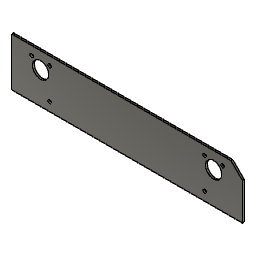
motor mount (Autodesk Fusion 360 design; units mm, degrees)
Autodesk Fusion 360 part; units mm, degrees
sketch "Sketch15" plane through (0, 0, 0) normal (0, 1, 0) x (1, 0, 0)
  line L0 (100, 21) -> (-100, 21)
  line L1 (-100, 21) -> (-100, -21)
  line L2 (-100, -21) -> (100, -21)
  line L3 (100, -21) -> (100, 21)
  line L4 (100, 21) -> (-100, -21) construction
  line L5 (-100, 21) -> (100, -21) construction
  dimension "d41" = 200
  dimension "d42" = 42
  constraint horizontal L0
  constraint perpendicular L0 L1
  constraint parallel L0 L2
  constraint parallel L1 L3
  constraint coincident L4 origin
  constraint coincident L5 origin
  measures "d41" distance of L1.end L2.end
  measures "d42" distance of L0.end L1.end
extrude "Extrude7" add sketch "Sketch15" along normal blind 1.5
hole "Hole5" at (67.2428, 0, 13.4085) direction (0, 1, 0) diameter 3 depth 7 tip angle 118
hole "Hole6" at (75.0009, 0, 6.5047) direction (0, 1, 0) diameter 14 depth 15 tip angle 118
hole "Hole7" at (82.7411, 0, 13.4378) direction (0, 1, 0) diameter 3 depth 5 tip angle 118
hole "Hole8" at (67.2952, 0, -13.4263) direction (0, 1, 0) diameter 3 depth 6 tip angle 118
sketch "Sketch16" plane through (0, 0, 0) normal (1, 0, 0) x (0, 1, 0)
  line L0 (-56.4532, 39.0008) -> (75, 39.0008)
  line L1 (75, 39.0008) -> (75, -35)
  line L2 (75, -35) -> (-56.4532, -35)
  line L3 (-56.4532, -35) -> (-56.4532, 39.0008)
  constraint horizontal L0
  constraint vertical L1
  constraint horizontal L2
  constraint vertical L3
ref_plane "WorkPlane2" through (0, 9.2734, 2.0004) normal (1, 0, 0) x (0, 1, 0)
mirror "Mirror1" about plane through (0, 9.2734, 2.0004) normal (1, 0, 0) of "Hole5", "Hole6", "Hole7", "Hole8"
chamfer "Chamfer1" distance 10 angle 45 1 edges at (100, 0.75, 21)
